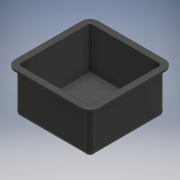
# Autodesk Inventor part: base
Saved by Autodesk Inventor 2017 (Build 210142000, 142)
## iProperties
Created: 2019-02-09
Part Number: base
Material: ABS Plastic
Document SubType Name: Modeling
Designer: felix
Density: 1.06 g/cm^3
Appearance: Smooth - Black
Author: felix
Autodesk Inventor part; units mm, degrees
ref_plane "YZ Plane" through (0, 0, 0) normal (1, 0, 0) x (0, 1, 0)
ref_plane "XZ Plane" through (0, 0, 0) normal (0, 1, 0) x (-1, 0, 0)
ref_plane "XY Plane" through (0, 0, 0) normal (0, 0, 1) x (1, 0, 0)
sketch "Sketch1" plane through (0, 0, 0) normal (0, 0, 1) x (1, 0, 0)
  line L0 (-39.5, -44.5) -> (39.5, -44.5)
  line L1 (44.5, -39.5) -> (44.5, 39.5)
  line L2 (39.5, 44.5) -> (-39.5, 44.5)
  line L3 (-44.5, 39.5) -> (-44.5, -39.5)
  line L4 (-44.5, -44.5) -> (44.5, 44.5) construction
  line L5 (44.5, -44.5) -> (-44.5, 44.5) construction
  arc A0 (-39.5, 44.5) -> (-44.5, 39.5) centre (-39.5, 39.5) ccw
  arc A1 (44.5, 39.5) -> (39.5, 44.5) centre (39.5, 39.5) ccw
  arc A2 (39.5, -44.5) -> (44.5, -39.5) centre (39.5, -39.5) ccw
  arc A3 (-44.5, -39.5) -> (-39.5, -44.5) centre (-39.5, -39.5) ccw
  line L6 (-39.5, 42.5) -> (39.5, 42.5)
  arc A4 (42.5, 39.5) -> (39.5, 42.5) centre (39.5, 39.5) ccw
  line L7 (42.5, 39.5) -> (42.5, -39.5)
  arc A5 (39.5, -42.5) -> (42.5, -39.5) centre (39.5, -39.5) ccw
  line L8 (39.5, -42.5) -> (-39.5, -42.5)
  arc A6 (-42.5, -39.5) -> (-39.5, -42.5) centre (-39.5, -39.5) ccw
  line L9 (-42.5, -39.5) -> (-42.5, 39.5)
  arc A7 (-39.5, 42.5) -> (-42.5, 39.5) centre (-39.5, 39.5) ccw
  line L10 (-49.5, -39.5) -> (-49.5, 39.5)
  arc A8 (-39.5, 49.5) -> (-49.5, 39.5) centre (-39.5, 39.5) ccw
  line L11 (-39.5, 49.5) -> (39.5, 49.5)
  arc A9 (49.5, 39.5) -> (39.5, 49.5) centre (39.5, 39.5) ccw
  line L12 (49.5, 39.5) -> (49.5, -39.5)
  arc A10 (39.5, -49.5) -> (49.5, -39.5) centre (39.5, -39.5) ccw
  line L13 (39.5, -49.5) -> (-39.5, -49.5)
  arc A11 (-49.5, -39.5) -> (-39.5, -49.5) centre (-39.5, -39.5) ccw
  point P0 (0, 0)
  dimension "d0" = 89
  dimension "d1" = 89
  dimension "d2" = 5
  dimension "d3" = 2
  dimension "d4" = 5
  constraints: 28 end point, 24 point on circle, 12 centre point, 8 point on line, 8 tangent, 6 parallel, 3 equal radius, 3 perpendicular, 2 midpoint, 1 horizontal, 14 other
  measures "d0" distance of L5.end L4.end
  measures "d1" distance of L4.end L5.start
  measures "d2" radius of A0
  measures "d3" distance between parallel lines of L2 L6
  measures "d4" distance between parallel lines of L3 L10
extrude "Extrusion1" add sketch "Sketch1" against normal blind 52 contours A3 L3 A0 L2 A1 L1 A2 L0 | L6 A4 L7 A5 L8 A6 L9 A7
extrude "Extrusion2" cut sketch "Sketch1" against normal blind 50 contours L6 A4 L7 A5 L8 A6 L9 A7
extrude "Extrusion3" add sketch "Sketch1" against normal blind 2 contours L10 A8 L11 A9 L12 A10 L13 A11
fillet "Fillet1" radius 5 8 edges at (43.0355, 43.0355, -52) (44.5, 0, -52) (43.0355, -43.0355, -52) (0, -44.5, -52) (-43.0355, -43.0355, -52) (-44.5, 0, -52) (-43.0355, 43.0355, -52) (0, 44.5, -52)
fillet "Fillet2" radius 3 8 edges at (-41.6213, -41.6213, -50) (-42.5, 0, -50) (-41.6213, 41.6213, -50) (0, 42.5, -50) (41.6213, 41.6213, -50) (42.5, 0, -50) (41.6213, -41.6213, -50) (0, -42.5, -50)
body "Solid1"
